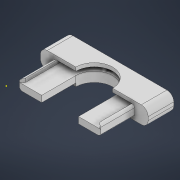
# Autodesk Inventor part: syringe_fitter
Saved by Autodesk Inventor 2022 (Build 260153000, 153)
## iProperties
Created: 2023-04-21
Part Number: syringe_fitter
Material: Generic
Document SubType Name: Modeling
Designer: Jakob Saugbjerg
Density: 1 g/cm^3
Appearance: Default
Author: Jakob Saugbjerg
Autodesk Inventor part; units mm, degrees
ref_plane "YZ Plane" through (0, 0, 0) normal (1, 0, 0) x (0, 1, 0)
ref_plane "XZ Plane" through (0, 0, 0) normal (0, 1, 0) x (-1, 0, 0)
ref_plane "XY Plane" through (0, 0, 0) normal (0, 0, 1) x (1, 0, 0)
sketch "Sketch13" plane through (0, 0, 0) normal (0, 0, 1) x (1, 0, 0)
  line L0 (0, 0) -> (63, 0)
  line L1 (63, 0) -> (63, 10)
  line L2 (63, 10) -> (0, 10)
  line L3 (0, 10) -> (0, 0)
  dimension "d38" = 63
  dimension "d39" = 10
  constraints: 8 end point, 2 parallel, 1 horizontal, 1 perpendicular
  measures "d38" distance of L2.end L1.end
  measures "d39" distance of L1.end L0.end
extrude "Extrusion8" add sketch "Sketch13" along normal blind 35
sketch "Sketch15" plane through (0, 10, 0) normal (0, 1, 0) x (1, 0, 0)
  line L0 (63, -35) -> (0, -35) projected
  line L1 (31.5, -35) -> (31.5, -15)
  circle A0 centre (31.5, -15) radius 10.75
  line L2 (44, -35) -> (20.75, -35)
  line L3 (20.75, -35) -> (20.75, -15)
  line L4 (42.25, -15) -> (42.25, -35)
  point P0 (0, 0)
  dimension "d42" = 20
  dimension "d43" = 21.5
  constraints: 8 end point, 2 point on circle, 2 point on line, 1 centre point, 1 coincident, 1 midpoint, 1 perpendicular, 1 vertical
  measures "d42" distance of L1.start L1.end
  measures "d43" diameter of A0
extrude "Extrusion9" cut sketch "Sketch15" against normal blind 35
sketch "Sketch16" plane through (0, 10, 0) normal (0, 1, 0) x (1, 0, 0)
  line L0 (0, -35) -> (20.75, -35) projected
  line L1 (0, -35) -> (63, -35)
  line L2 (63, -35) -> (63, -15)
  line L3 (63, -15) -> (0, -15)
  line L4 (0, -15) -> (0, -35)
  point P0 (0, 0)
  dimension "d46" = 63
  dimension "d47" = 20
  constraints: 8 end point, 2 parallel, 1 horizontal, 1 perpendicular
  measures "d46" distance of L3.end L2.end
  measures "d47" distance of L2.end L1.end
extrude "Extrusion10" cut sketch "Sketch16" against normal blind 2.1
sketch "Sketch17" plane through (0, 0, 0) normal (0, -1, 0) x (1, 0, 0)
  line L0 (0, 0) -> (0, 35) projected
  line L1 (63, 15) -> (63, 35) projected
  line L2 (0, 35) -> (63, 35)
  line L3 (63, 35) -> (63, 15)
  line L4 (63, 15) -> (0, 15)
  line L5 (0, 15) -> (0, 35)
  dimension "d50" = 20
  constraints: 8 end point, 2 parallel, 1 horizontal, 1 perpendicular
  measures "d50" distance of L2.end L1.start
extrude "Extrusion11" cut sketch "Sketch17" against normal blind 2
sketch "Sketch19" plane through (0, 0, 35) normal (0, 0, 1) x (1, 0, 0)
  line L0 (20.75, 7.9) -> (0, 7.9) projected
  line L1 (9.5, 7.9) -> (53.5, 7.9)
  line L2 (53.5, 7.9) -> (53.5, 5.7)
  line L3 (53.5, 5.7) -> (9.5, 5.7)
  line L4 (9.5, 5.7) -> (9.5, 7.9)
  point P0 (0, 0)
  point P1 (31.5, 5.25)
  dimension "d68" = 2.2
  constraints: 8 end point, 2 parallel, 1 horizontal, 1 perpendicular, 1 point on line
  measures "d68" distance of L1.end L2.end
extrude "Extrusion12" cut sketch "Sketch19" against normal blind 33
fillet "Fillet5" radius 2 2 edges at (9.5, 6.8, 35) (53.5, 6.8, 35)
sketch "Sketch20" plane through (0, 0, 35) normal (0, 0, 1) x (1, 0, 0)
  line L0 (63, 7.9) -> (42.25, 7.9) projected
  line L1 (7.5, 1.9) -> (55.5, 1.9)
  line L2 (55.5, 1.9) -> (55.5, 7.9)
  line L3 (55.5, 7.9) -> (7.5, 7.9)
  line L4 (7.5, 7.9) -> (7.5, 1.9)
  line L5 (7.5, 1.9) -> (55.5, 7.9) construction
  line L6 (55.5, 1.9) -> (7.5, 7.9) construction
  line L7 (7.5, 7.9) -> (0, 7.9)
  line L8 (0, 7.9) -> (0, 1.9)
  line L9 (0, 1.9) -> (7.5, 1.9)
  line L10 (7.5, 1.9) -> (7.5, 7.9)
  line L11 (42.25, 2) -> (63, 2) projected
  line L12 (55.5, 7.9) -> (63, 7.9)
  line L13 (63, 7.9) -> (63, 2)
  line L14 (63, 2) -> (55.5, 2)
  line L15 (55.5, 2) -> (55.5, 7.9)
  point P0 (0, 0)
  point P1 (31.5, 4.9)
  point P2 (55.5, 2)
  dimension "d58" = 48
  constraints: 26 end point, 5 parallel, 3 horizontal, 2 midpoint, 2 perpendicular, 1 point on line, 1 vertical, 4 other
  measures "d58" distance of L3.end L2.end
extrude "Extrusion13" cut sketch "Sketch20" against normal blind 20 contours L13 L11 L2 L0 | L4 L9 L8 L7
fillet "Fillet6" radius 2 4 edges at (7.5, 7.9, 25) (7.5, 2, 25) (55.5, 7.9, 25) (55.5, 2, 25)
sketch "Sketch21" plane through (0, 0, 0) normal (0, 0, -1) x (-1, 0, 0)
  line L0 (-42.2521, 3.6325) -> (-44.1318, 3.6325)
  line L1 (-44.1318, 3.6325) -> (-44.1318, 4.0648)
  spline S0 degree 2 poles (-44.1318, 4.0648) (-43.9292, 4.255) (-43.5686, 4.6082) (-43.3957, 4.7984) knots 0 0 0 1 2 2 2
  spline S1 degree 2 poles (-43.3957, 4.7984) (-43.0474, 5.1812) (-42.793, 5.6407) (-42.793, 5.8852) knots 0 0 0 1 2 2 2
  spline S2 degree 2 poles (-42.793, 5.8852) (-42.793, 6.0136) (-42.8721, 6.2063) (-42.9437, 6.268) knots 0 0 0 1 2 2 2
  spline S3 degree 2 poles (-42.9437, 6.268) (-43.0153, 6.3298) (-43.2031, 6.3915) (-43.3167, 6.3915) knots 0 0 0 1 2 2 2
  spline S4 degree 2 poles (-43.3167, 6.3915) (-43.4254, 6.3915) (-43.6477, 6.3372) (-43.7489, 6.2952) knots 0 0 0 1 2 2 2
  spline S5 degree 2 poles (-43.7489, 6.2952) (-43.8354, 6.2606) (-43.9959, 6.1618) (-44.0453, 6.1272) knots 0 0 0 1 2 2 2
  line L2 (-44.0453, 6.1272) -> (-44.0676, 6.1272)
  line L3 (-44.0676, 6.1272) -> (-44.0676, 6.562)
  spline S6 degree 2 poles (-44.0676, 6.562) (-43.9416, 6.6237) (-43.4896, 6.7448) (-43.287, 6.7448) knots 0 0 0 1 2 2 2
  spline S7 degree 2 poles (-43.287, 6.7448) (-42.8597, 6.7448) (-42.3781, 6.2927) (-42.3781, 5.9074) knots 0 0 0 1 2 2 2
  spline S8 degree 2 poles (-42.3781, 5.9074) (-42.3781, 5.7271) (-42.4621, 5.4258) (-42.5362, 5.2973) knots 0 0 0 1 2 2 2
  spline S9 degree 2 poles (-42.5362, 5.2973) (-42.6103, 5.1639) (-42.8251, 4.9021) (-42.9437, 4.7762) knots 0 0 0 1 2 2 2
  spline S10 degree 2 poles (-42.9437, 4.7762) (-43.1364, 4.5662) (-43.6081, 4.1167) (-43.7489, 3.9857) knots 0 0 0 1 2 2 2
  line L4 (-43.7489, 3.9857) -> (-42.2521, 3.9857)
  line L5 (-42.2521, 3.9857) -> (-42.2521, 3.6325)
  spline S11 degree 2 poles (-39.9476, 5.1565) (-39.9476, 4.3365) (-40.4243, 3.5683) (-40.9208, 3.5683) knots 0 0 0 1 2 2 2
  spline S12 degree 2 poles (-40.9208, 3.5683) (-41.4246, 3.5683) (-41.8964, 4.3513) (-41.8964, 5.1541) knots 0 0 0 1 2 2 2
  spline S13 degree 2 poles (-41.8964, 5.1541) (-41.8964, 5.979) (-41.4197, 6.7423) (-40.9208, 6.7423) knots 0 0 0 1 2 2 2
  spline S14 degree 2 poles (-40.9208, 6.7423) (-40.4194, 6.7423) (-39.9476, 5.9519) (-39.9476, 5.1565) knots 0 0 0 1 2 2 2
  spline S15 degree 2 poles (-40.4712, 4.2278) (-40.4119, 4.3785) (-40.3625, 4.8428) (-40.3625, 5.1565) knots 0 0 0 1 2 2 2
  spline S16 degree 2 poles (-40.3625, 5.1565) (-40.3625, 5.4702) (-40.4119, 5.9321) (-40.4737, 6.0877) knots 0 0 0 1 2 2 2
  spline S17 degree 2 poles (-40.4737, 6.0877) (-40.5354, 6.2433) (-40.7503, 6.4039) (-40.9208, 6.4039) knots 0 0 0 1 2 2 2
  spline S18 degree 2 poles (-40.9208, 6.4039) (-41.0912, 6.4039) (-41.311, 6.2433) (-41.3752, 6.0828) knots 0 0 0 1 2 2 2
  spline S19 degree 2 poles (-41.3752, 6.0828) (-41.437, 5.9272) (-41.4815, 5.4529) (-41.4815, 5.1541) knots 0 0 0 1 2 2 2
  spline S20 degree 2 poles (-41.4815, 5.1541) (-41.4815, 4.833) (-41.4419, 4.4032) (-41.3777, 4.2352) knots 0 0 0 1 2 2 2
  spline S21 degree 2 poles (-41.3777, 4.2352) (-41.3184, 4.0771) (-41.0986, 3.9067) (-40.9208, 3.9067) knots 0 0 0 1 2 2 2
  spline S22 degree 2 poles (-40.9208, 3.9067) (-40.7528, 3.9067) (-40.533, 4.0673) (-40.4712, 4.2278) knots 0 0 0 1 2 2 2
  line L6 (-35.5979, 3.6325) -> (-35.5979, 4.9565)
  spline S23 degree 2 poles (-35.5979, 4.9565) (-35.5979, 5.1145) (-35.6226, 5.3838) (-35.6621, 5.4579) knots 0 0 0 1 2 2 2
  spline S24 degree 2 poles (-35.6621, 5.4579) (-35.7016, 5.5394) (-35.8523, 5.6184) (-35.9832, 5.6184) knots 0 0 0 1 2 2 2
  spline S25 degree 2 poles (-35.9832, 5.6184) (-36.1018, 5.6184) (-36.3735, 5.4727) (-36.5167, 5.3344) knots 0 0 0 1 2 2 2
  spline S26 degree 2 poles (-36.5167, 5.3344) (-36.5143, 5.2998) (-36.5093, 5.2035) (-36.5093, 5.1392) knots 0 0 0 1 2 2 2
  line L7 (-36.5093, 5.1392) -> (-36.5093, 3.6325)
  line L8 (-36.5093, 3.6325) -> (-36.8946, 3.6325)
  line L9 (-36.8946, 3.6325) -> (-36.8946, 4.9565)
  spline S27 degree 2 poles (-36.8946, 4.9565) (-36.8946, 5.1145) (-36.9193, 5.3838) (-36.9589, 5.4579) knots 0 0 0 1 2 2 2
  spline S28 degree 2 poles (-36.9589, 5.4579) (-36.9984, 5.5394) (-37.1491, 5.6184) (-37.28, 5.6184) knots 0 0 0 1 2 2 2
  spline S29 degree 2 poles (-37.28, 5.6184) (-37.4035, 5.6184) (-37.6776, 5.4628) (-37.8061, 5.3418) knots 0 0 0 1 2 2 2
  line L10 (-37.8061, 5.3418) -> (-37.8061, 3.6325)
  line L11 (-37.8061, 3.6325) -> (-38.1914, 3.6325)
  line L12 (-38.1914, 3.6325) -> (-38.1914, 5.9198)
  line L13 (-38.1914, 5.9198) -> (-37.8061, 5.9198)
  line L14 (-37.8061, 5.9198) -> (-37.8061, 5.6678)
  spline S30 degree 2 poles (-37.8061, 5.6678) (-37.6554, 5.8185) (-37.359, 5.984) (-37.1812, 5.984) knots 0 0 0 1 2 2 2
  spline S31 degree 2 poles (-37.1812, 5.984) (-36.9786, 5.984) (-36.6649, 5.7987) (-36.5834, 5.5888) knots 0 0 0 1 2 2 2
  spline S32 degree 2 poles (-36.5834, 5.5888) (-36.408, 5.7839) (-36.0771, 5.984) (-35.8844, 5.984) knots 0 0 0 1 2 2 2
  spline S33 degree 2 poles (-35.8844, 5.984) (-35.7362, 5.984) (-35.4941, 5.8926) (-35.4052, 5.7889) knots 0 0 0 1 2 2 2
  spline S34 degree 2 poles (-35.4052, 5.7889) (-35.3138, 5.6851) (-35.2126, 5.3739) (-35.2126, 5.1392) knots 0 0 0 1 2 2 2
  line L15 (-35.2126, 5.1392) -> (-35.2126, 3.6325)
  line L16 (-35.2126, 3.6325) -> (-35.5979, 3.6325)
  line L17 (-32.8759, 3.6325) -> (-34.642, 3.6325)
  line L18 (-34.642, 3.6325) -> (-34.642, 6.6805)
  line L19 (-34.642, 6.6805) -> (-34.2369, 6.6805)
  line L20 (-34.2369, 6.6805) -> (-34.2369, 3.9932)
  line L21 (-34.2369, 3.9932) -> (-32.8759, 3.9932)
  line L22 (-32.8759, 3.9932) -> (-32.8759, 3.6325)
  spline S35 degree 2 poles (-30.6603, 3.5782) (-30.89, 3.5782) (-31.2877, 3.7017) (-31.4186, 3.7709) knots 0 0 0 1 2 2 2
  line L23 (-31.4186, 3.7709) -> (-31.4186, 4.2031)
  line L24 (-31.4186, 4.2031) -> (-31.3989, 4.2031)
  spline S36 degree 2 poles (-31.3989, 4.2031) (-31.3495, 4.1636) (-31.2161, 4.0697) (-31.1049, 4.0179) knots 0 0 0 1 2 2 2
  spline S37 degree 2 poles (-31.1049, 4.0179) (-31.0086, 3.9709) (-30.7715, 3.9018) (-30.6455, 3.9018) knots 0 0 0 1 2 2 2
  spline S38 degree 2 poles (-30.6455, 3.9018) (-30.5541, 3.9018) (-30.3442, 3.9438) (-30.2948, 3.9783) knots 0 0 0 1 2 2 2
  spline S39 degree 2 poles (-30.2948, 3.9783) (-30.2231, 4.0253) (-30.1589, 4.1315) (-30.1589, 4.2402) knots 0 0 0 1 2 2 2
  spline S40 degree 2 poles (-30.1589, 4.2402) (-30.1589, 4.376) (-30.3071, 4.5168) (-30.4973, 4.5637) knots 0 0 0 1 2 2 2
  spline S41 degree 2 poles (-30.4973, 4.5637) (-30.5714, 4.581) (-30.8085, 4.6304) (-30.9098, 4.6576) knots 0 0 0 1 2 2 2
  spline S42 degree 2 poles (-30.9098, 4.6576) (-31.1716, 4.7342) (-31.4087, 5.0503) (-31.4087, 5.2751) knots 0 0 0 1 2 2 2
  spline S43 degree 2 poles (-31.4087, 5.2751) (-31.4087, 5.5863) (-30.9419, 5.9741) (-30.5566, 5.9741) knots 0 0 0 1 2 2 2
  spline S44 degree 2 poles (-30.5566, 5.9741) (-30.3664, 5.9741) (-29.9811, 5.8802) (-29.8502, 5.8086) knots 0 0 0 1 2 2 2
  line L25 (-29.8502, 5.8086) -> (-29.8502, 5.3961)
  line L26 (-29.8502, 5.3961) -> (-29.8699, 5.3961)
  spline S45 degree 2 poles (-29.8699, 5.3961) (-30.0181, 5.5147) (-30.3787, 5.6505) (-30.564, 5.6505) knots 0 0 0 1 2 2 2
  spline S46 degree 2 poles (-30.564, 5.6505) (-30.7542, 5.6505) (-31.016, 5.49) (-31.016, 5.3294) knots 0 0 0 1 2 2 2
  spline S47 degree 2 poles (-31.016, 5.3294) (-31.016, 5.1837) (-30.8604, 5.0429) (-30.6875, 4.9985) knots 0 0 0 1 2 2 2
  spline S48 degree 2 poles (-30.6875, 4.9985) (-30.6035, 4.9762) (-30.3911, 4.9318) (-30.275, 4.9046) knots 0 0 0 1 2 2 2
  spline S49 degree 2 poles (-30.275, 4.9046) (-30.0231, 4.8404) (-29.7662, 4.5464) (-29.7662, 4.292) knots 0 0 0 1 2 2 2
  spline S50 degree 2 poles (-29.7662, 4.292) (-29.7662, 4.1438) (-29.8823, 3.882) (-29.9959, 3.7857) knots 0 0 0 1 2 2 2
  spline S51 degree 2 poles (-29.9959, 3.7857) (-30.1169, 3.6844) (-30.4257, 3.5782) (-30.6603, 3.5782) knots 0 0 0 1 2 2 2
  line L27 (-27.6123, 5.9198) -> (-28.8424, 2.7903)
  line L28 (-28.8424, 2.7903) -> (-29.2549, 2.7903)
  line L29 (-29.2549, 2.7903) -> (-28.8449, 3.7437)
  line L30 (-28.8449, 3.7437) -> (-29.6748, 5.9198)
  line L31 (-29.6748, 5.9198) -> (-29.2598, 5.9198)
  line L32 (-29.2598, 5.9198) -> (-28.6349, 4.2253)
  line L33 (-28.6349, 4.2253) -> (-28.0125, 5.9198)
  line L34 (-28.0125, 5.9198) -> (-27.6123, 5.9198)
  line L35 (-26.1081, 5.5073) -> (-26.1278, 5.5073)
  spline S52 degree 2 poles (-26.1278, 5.5073) (-26.1723, 5.5196) (-26.2686, 5.5246) (-26.3353, 5.5246) knots 0 0 0 1 2 2 2
  spline S53 degree 2 poles (-26.3353, 5.5246) (-26.4909, 5.5246) (-26.7972, 5.3887) (-26.9355, 5.2553) knots 0 0 0 1 2 2 2
  line L36 (-26.9355, 5.2553) -> (-26.9355, 3.6325)
  line L37 (-26.9355, 3.6325) -> (-27.3209, 3.6325)
  line L38 (-27.3209, 3.6325) -> (-27.3209, 5.9198)
  line L39 (-27.3209, 5.9198) -> (-26.9355, 5.9198)
  line L40 (-26.9355, 5.9198) -> (-26.9355, 5.5789)
  spline S54 degree 2 poles (-26.9355, 5.5789) (-26.7256, 5.7666) (-26.4119, 5.9198) (-26.2637, 5.9198) knots 0 0 0 1 2 2 2
  spline S55 degree 2 poles (-26.2637, 5.9198) (-26.2044, 5.9198) (-26.1451, 5.9148) (-26.1081, 5.9074) knots 0 0 0 1 2 2 2
  line L41 (-26.1081, 5.9074) -> (-26.1081, 5.5073)
  line L42 (-25.4165, 3.6325) -> (-25.8018, 3.6325)
  line L43 (-25.8018, 3.6325) -> (-25.8018, 5.9198)
  line L44 (-25.8018, 5.9198) -> (-25.4165, 5.9198)
  line L45 (-25.4165, 5.9198) -> (-25.4165, 3.6325)
  line L46 (-25.3893, 6.3002) -> (-25.8265, 6.3002)
  line L47 (-25.8265, 6.3002) -> (-25.8265, 6.7003)
  line L48 (-25.8265, 6.7003) -> (-25.3893, 6.7003)
  line L49 (-25.3893, 6.7003) -> (-25.3893, 6.3002)
  line L50 (-23.0551, 3.6325) -> (-23.4405, 3.6325)
  line L51 (-23.4405, 3.6325) -> (-23.4405, 4.9367)
  spline S56 degree 2 poles (-23.4405, 4.9367) (-23.4405, 5.0948) (-23.4701, 5.3665) (-23.5146, 5.448) knots 0 0 0 1 2 2 2
  spline S57 degree 2 poles (-23.5146, 5.448) (-23.5615, 5.5344) (-23.7295, 5.6184) (-23.8727, 5.6184) knots 0 0 0 1 2 2 2
  spline S58 degree 2 poles (-23.8727, 5.6184) (-24.016, 5.6184) (-24.3198, 5.4653) (-24.4655, 5.3418) knots 0 0 0 1 2 2 2
  line L52 (-24.4655, 5.3418) -> (-24.4655, 3.6325)
  line L53 (-24.4655, 3.6325) -> (-24.8508, 3.6325)
  line L54 (-24.8508, 3.6325) -> (-24.8508, 5.9198)
  line L55 (-24.8508, 5.9198) -> (-24.4655, 5.9198)
  line L56 (-24.4655, 5.9198) -> (-24.4655, 5.6654)
  spline S59 degree 2 poles (-24.4655, 5.6654) (-24.2926, 5.821) (-23.9592, 5.984) (-23.7714, 5.984) knots 0 0 0 1 2 2 2
  spline S60 degree 2 poles (-23.7714, 5.984) (-23.4355, 5.984) (-23.0551, 5.5394) (-23.0551, 5.117) knots 0 0 0 1 2 2 2
  line L57 (-23.0551, 5.117) -> (-23.0551, 3.6325)
  spline S61 degree 2 poles (-22.4327, 3.267) (-22.3932, 3.2497) (-22.2425, 3.1953) (-22.1462, 3.1731) knots 0 0 0 1 2 2 2
  spline S62 degree 2 poles (-22.1462, 3.1731) (-22.04, 3.1459) (-21.8596, 3.1138) (-21.7534, 3.1138) knots 0 0 0 1 2 2 2
  spline S63 degree 2 poles (-21.7534, 3.1138) (-21.5756, 3.1138) (-21.3286, 3.2077) (-21.2594, 3.2917) knots 0 0 0 1 2 2 2
  spline S64 degree 2 poles (-21.2594, 3.2917) (-21.1927, 3.3757) (-21.1409, 3.5955) (-21.1409, 3.7363) knots 0 0 0 1 2 2 2
  line L58 (-21.1409, 3.7363) -> (-21.1409, 3.9363)
  spline S65 degree 2 poles (-21.1409, 3.9363) (-21.2965, 3.8005) (-21.5954, 3.6721) (-21.8201, 3.6721) knots 0 0 0 1 2 2 2
  spline S66 degree 2 poles (-21.8201, 3.6721) (-22.2104, 3.6721) (-22.6723, 4.2525) (-22.6723, 4.7984) knots 0 0 0 1 2 2 2
  spline S67 degree 2 poles (-22.6723, 4.7984) (-22.6723, 5.0824) (-22.5117, 5.5221) (-22.3784, 5.6777) knots 0 0 0 1 2 2 2
  spline S68 degree 2 poles (-22.3784, 5.6777) (-22.2499, 5.8234) (-21.8967, 5.984) (-21.709, 5.984) knots 0 0 0 1 2 2 2
  spline S69 degree 2 poles (-21.709, 5.984) (-21.5311, 5.984) (-21.2718, 5.9) (-21.1409, 5.8234) knots 0 0 0 1 2 2 2
  line L59 (-21.1409, 5.8234) -> (-21.1186, 5.9198)
  line L60 (-21.1186, 5.9198) -> (-20.7556, 5.9198)
  line L61 (-20.7556, 5.9198) -> (-20.7556, 3.8944)
  spline S70 degree 2 poles (-20.7556, 3.8944) (-20.7556, 3.3114) (-21.2619, 2.768) (-21.7831, 2.768) knots 0 0 0 1 2 2 2
  spline S71 degree 2 poles (-21.7831, 2.768) (-21.951, 2.768) (-22.3018, 2.8224) (-22.4525, 2.8668) knots 0 0 0 1 2 2 2
  line L62 (-22.4525, 2.8668) -> (-22.4525, 3.267)
  line L63 (-22.4525, 3.267) -> (-22.4327, 3.267)
  line L64 (-21.1409, 4.2525) -> (-21.1409, 5.5097)
  spline S72 degree 2 poles (-21.1409, 5.5097) (-21.2841, 5.5789) (-21.5262, 5.6382) (-21.6472, 5.6382) knots 0 0 0 1 2 2 2
  spline S73 degree 2 poles (-21.6472, 5.6382) (-21.9387, 5.6382) (-22.2746, 5.2084) (-22.2746, 4.8058) knots 0 0 0 1 2 2 2
  spline S74 degree 2 poles (-22.2746, 4.8058) (-22.2746, 4.4254) (-22.0202, 4.0277) (-21.7337, 4.0277) knots 0 0 0 1 2 2 2
  spline S75 degree 2 poles (-21.7337, 4.0277) (-21.583, 4.0277) (-21.2668, 4.1463) (-21.1409, 4.2525) knots 0 0 0 1 2 2 2
  spline S76 degree 2 poles (-19.2044, 3.5807) (-19.7527, 3.5807) (-20.3554, 4.1957) (-20.3554, 4.7638) knots 0 0 0 1 2 2 2
  spline S77 degree 2 poles (-20.3554, 4.7638) (-20.3554, 5.322) (-19.77, 5.984) (-19.2982, 5.984) knots 0 0 0 1 2 2 2
  spline S78 degree 2 poles (-19.2982, 5.984) (-19.0858, 5.984) (-18.7573, 5.8605) (-18.6363, 5.7296) knots 0 0 0 1 2 2 2
  spline S79 degree 2 poles (-18.6363, 5.7296) (-18.5128, 5.5987) (-18.3819, 5.2208) (-18.3819, 4.9466) knots 0 0 0 1 2 2 2
  line L65 (-18.3819, 4.9466) -> (-18.3819, 4.7366)
  line L66 (-18.3819, 4.7366) -> (-19.9651, 4.7366)
  spline S80 degree 2 poles (-19.9651, 4.7366) (-19.9651, 4.339) (-19.565, 3.9166) (-19.2093, 3.9166) knots 0 0 0 1 2 2 2
  spline S81 degree 2 poles (-19.2093, 3.9166) (-19.0834, 3.9166) (-18.8388, 3.9734) (-18.74, 4.0179) knots 0 0 0 1 2 2 2
  spline S82 degree 2 poles (-18.74, 4.0179) (-18.6363, 4.0673) (-18.493, 4.1537) (-18.4461, 4.1932) knots 0 0 0 1 2 2 2
  line L67 (-18.4461, 4.1932) -> (-18.4239, 4.1932)
  line L68 (-18.4239, 4.1932) -> (-18.4239, 3.7733)
  spline S83 degree 2 poles (-18.4239, 3.7733) (-18.4905, 3.7462) (-18.6931, 3.6671) (-18.7721, 3.6449) knots 0 0 0 1 2 2 2
  spline S84 degree 2 poles (-18.7721, 3.6449) (-18.8833, 3.6128) (-19.0661, 3.5807) (-19.2044, 3.5807) knots 0 0 0 1 2 2 2
  spline S85 degree 2 poles (-18.7573, 5.0306) (-18.7622, 5.1862) (-18.8265, 5.4134) (-18.8882, 5.49) knots 0 0 0 1 2 2 2
  spline S86 degree 2 poles (-18.8882, 5.49) (-18.9549, 5.5764) (-19.1649, 5.6678) (-19.3205, 5.6678) knots 0 0 0 1 2 2 2
  spline S87 degree 2 poles (-19.3205, 5.6678) (-19.4736, 5.6678) (-19.6885, 5.5764) (-19.7774, 5.4875) knots 0 0 0 1 2 2 2
  spline S88 degree 2 poles (-19.7774, 5.4875) (-19.8639, 5.3961) (-19.9528, 5.1763) (-19.9651, 5.0306) knots 0 0 0 1 2 2 2
  line L69 (-19.9651, 5.0306) -> (-18.7573, 5.0306)
  point P0 (0, 0)
  point P1 (-44.3541, 6.7448)
  dimension "d39" = 10
  constraints: 1 other
emboss "Emboss3" sketch "Sketch21" operation cut depth 1 direction (0, 0, 1)
sketch "Sketch22" plane through (0, 0, 35) normal (0, 0, 1) x (1, 0, 0)
  point P0 (0, 0)
sketch "Sketch23" plane through (55.5, 4, 15) normal (1, 0, 0) x (0, 0, -1)
  line L0 (0, 3.8) -> (-20, 3.8) projected
  line L1 (-20, -2) -> (0, -2) projected
  line L2 (-20, 3.8) -> (0, 3.8)
  line L3 (0, 3.8) -> (0, -2)
  line L4 (0, -2) -> (-20, -2)
  line L5 (-20, -2) -> (-20, 3.8)
  point P0 (15, -4)
  constraints: 8 end point, 2 parallel, 1 horizontal, 1 perpendicular
extrude "Extrusion14" cut sketch "Sketch23" against normal blind 0.2
sketch "Sketch24" plane through (7.5, 4, 15) normal (-1, 0, 0) x (0, 0, 1)
  line L0 (20, 2.25) -> (20, 1.9) projected
  line L1 (20, -2) -> (0, -2) projected
  line L2 (20, 2.25) -> (0, 2.25)
  line L3 (0, 2.25) -> (0, -2)
  line L4 (0, -2) -> (20, -2)
  line L5 (20, -2) -> (20, 2.25)
  line L6 (0, 1.7) -> (0, -2) projected
  line L7 (0, 2.25) -> (20, 2.25)
  line L8 (20, 2.25) -> (20, 4.4148)
  line L9 (20, 4.4148) -> (0, 4.4148)
  line L10 (0, 4.4148) -> (0, 2.25)
  point P0 (-15, -4)
  constraints: 16 end point, 4 parallel, 2 horizontal, 2 perpendicular
extrude "Extrusion15" cut sketch "Sketch24" against normal blind 0.2
fillet "Fillet7" radius 4 4 edges at (0, 10, 7.5) (0, 0, 7.5) (63, 10, 7.5) (63, 0, 7.5)
sketch "Sketch25" plane through (0, 0, 35) normal (0, 0, 1) x (1, 0, 0)
  point P0 (0, 0)
body "Solid2"
